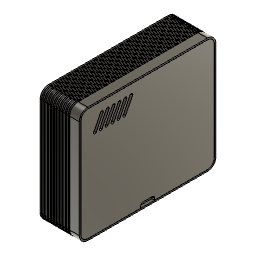
co2sensor_case (Autodesk Fusion 360 design; units mm, degrees)
Autodesk Fusion 360 part; units mm, degrees
note: some values were not read from the file. Set by a fixed rule: which sketch regions a step uses.
sketch "Front Layout" plane through (0, 0, 0) normal (1, 0, 0) x (0, 1, 0) in component "Front"
  line L0 (0, 0) -> (-45.7, 0)
  line L1 (-45.7, 0) -> (-45.7, 77.4)
  line L2 (-45.7, 77.4) -> (0, 77.4)
  line L3 (0, 77.4) -> (0, 0)
  line L4 (-48.7, 80.4) -> (0, 80.4)
  line L5 (0, 80.4) -> (0, -2)
  line L6 (0, -2) -> (-48.7, -2)
  line L7 (-48.7, -2) -> (-48.7, 80.4)
  line L8 (-42.2, 73.9) -> (0, 73.9)
  line L9 (0, 73.9) -> (0, 10.5)
  line L10 (0, 10.5) -> (-42.2, 10.5)
  line L11 (-42.2, 10.5) -> (-42.2, 73.9)
  dimension "d43" = 45.7
  dimension "d44" = 77.4
  dimension "d45" = 3
  dimension "d46" = 3
  dimension "d47" = 2
  dimension "d48" = 3.5
  dimension "d49" = 3.5
  dimension "d50" = 10.5
  constraint horizontal L0
  constraint vertical L1
  constraint horizontal L2
  constraint vertical L3
  constraint coincident L0.start L3.end
  constraint horizontal L4
  constraint vertical L5
  constraint horizontal L6
  constraint vertical L7
  constraint collinear L3 L5
  constraint horizontal L8
  constraint vertical L9
  constraint horizontal L10
  constraint vertical L11
  constraint collinear L3 L9
  measures "d43" distance of L0.start L0.end
  measures "d44" distance of L0.start L2.end
  measures "d45" distance of L2 L4
  measures "d46" distance of L1 L7
  measures "d47" distance of L0 L6
  measures "d48" distance of L2 L8
  measures "d49" distance of L1 L11
  measures "d50" distance of L0 L10
extrude "Extrude5" add sketch "Front Layout" along normal blind 28 makes body 1 in component "Front"
fillet "Fillet4" radius 6 2 edges at (14, -48.7, 80.4) (14, -48.7, -2) on bodies 1 in component "Front"
shell "Shell2" thickness 3 removed faces 2 at (18.6667, 0, 52.9333) at (28, -16.2333, 50.9333) on bodies 1 in component "Front"
extrude "Extrude6" cut sketch "Front Layout" along normal blind 3 contours L3 L5 L8 L9 L10 L11 bodies 1 in component "Front"
fillet "Fillet5" radius 3 2 edges at (1.5, -42.2, 73.9) (1.5, -42.2, 10.5) on bodies 1 in component "Front"
extrude "Extrude7" cut sketch "Front Layout" along normal blind 60 from surface at 3 contours L0 L1 L2 L3 L5 L8 L10 L11 bodies 1 in component "Front"
extrude "Extrude8" cut 1 faces at (3, -28.3, 3.5) along direction (-1, 0, 0) blind 1 on bodies 1 bodies 1 in component "Front"
sketch "Case Ribs" plane through (0, 0, 0) normal (-1, 0, 0) x (0, -1, 0) in component "Front"
  line L0 (39.2, 10.5) -> (0, 10.5)
  line L1 (0, 10.5) -> (0, -2)
  line L2 (0, -2) -> (42.7, -2)
  arc A0 (42.7, -2) -> (48.7, 4) centre (42.7, 4) ccw
  line L3 (48.7, 4) -> (48.7, 74.4)
  arc A1 (48.7, 74.4) -> (42.7, 80.4) centre (42.7, 74.4) ccw
  line L4 (42.7, 80.4) -> (0, 80.4)
  line L5 (0, 80.4) -> (0, 73.9)
  line L6 (0, 73.9) -> (39.2, 73.9)
  arc A2 (42.2, 70.9) -> (39.2, 73.9) centre (39.2, 70.9) ccw
  line L7 (42.2, 70.9) -> (42.2, 13.5)
  arc A3 (39.2, 10.5) -> (42.2, 13.5) centre (39.2, 13.5) ccw
  line L8 (0, -1.8) -> (42.7, -1.8)
  arc A4 (42.7, -1.8) -> (48.5, 4) centre (42.7, 4) ccw
  line L9 (48.5, 4) -> (48.5, 74.4)
  arc A5 (48.5, 74.4) -> (42.7, 80.2) centre (42.7, 74.4) ccw
  line L10 (42.7, 80.2) -> (0, 80.2)
  dimension "d67" = -0.2
extrude "Extrude9" cut sketch "Case Ribs" along normal blind 1 from surface at -2 contours L1 L2 A0 L3 A1 L4 L5 L8 A4 L9 A5 L10 bodies 1 in component "Front"
pattern_linear "R-Pattern1" count 10 spacing 2.1111 along (1, 0, 0) of "Extrude9" in component "Front"
sketch "Inlay Tabs" plane through (0, -45.7, 0) normal (0, 1, 0) x (-1, 0, 0) in component "Front"
  line L0 (-2, 77.4) -> (-28, 77.4)
  line L1 (-28, 77.4) -> (-28, 0)
  line L2 (-28, 0) -> (-2, 0)
  line L3 (-2, 0) -> (-2, 77.4)
  line L4 (-28, 71.4) -> (-2, 71.4)
  line L5 (-2, 71.4) -> (-2, 59.4)
  line L6 (-2, 59.4) -> (-28, 59.4)
  line L7 (-28, 59.4) -> (-28, 71.4)
  line L8 (-28, 18) -> (-2, 18)
  line L9 (-2, 18) -> (-2, 6)
  line L10 (-2, 6) -> (-28, 6)
  line L11 (-28, 6) -> (-28, 18)
  line L12 (-2, 70.9) -> (-2, 13.5)
  line L13 (-28, 77.4) -> (-2, 77.4)
  line L14 (-2, 0) -> (-28, 0)
  dimension "d81" = 12
  dimension "d82" = 12
  dimension "d83" = 6
  dimension "d84" = 6
  constraint horizontal L4
  constraint vertical L5
  constraint horizontal L6
  constraint vertical L7
  constraint horizontal L8
  constraint vertical L9
  constraint horizontal L10
  constraint vertical L11
  constraint collinear L5 L12
  constraint collinear L3 L9
  constraint collinear L1 L11
  constraint collinear L1 L7
  measures "d81" distance of L4.start L6.end
  measures "d82" distance of L8.start L10.end
  measures "d83" distance of L4 L13
  measures "d84" distance of L10 L14
extrude "Extrude11" cut sketch "Inlay Tabs" against normal blind 1 contours L1 L3 L4 L5 L6 L7 L12 | L1 L3 L8 L9 L10 L11 L12 bodies 1 in component "Front"
sketch "Backplate Groove" plane through (28, 0, 0) normal (1, 0, 0) x (0, 1, 0) in component "Front"
  line L0 (-45.7, 71.4) -> (-45.7, 77.4)
  line L1 (-45.7, 77.4) -> (0, 77.4)
  line L2 (0, 77.4) -> (0, 80.4)
  line L3 (0, 80.4) -> (-42.7, 80.4)
  arc A0 (-42.7, 80.4) -> (-48.7, 74.4) centre (-42.7, 74.4) ccw
  line L4 (-48.7, 74.4) -> (-48.7, 4)
  arc A1 (-48.7, 4) -> (-42.7, -2) centre (-42.7, 4) ccw
  line L5 (-42.7, -2) -> (0, -2)
  line L6 (0, -2) -> (0, 0)
  line L7 (0, 79.4) -> (-42.7, 79.4)
  arc A2 (-42.7, 79.4) -> (-47.7, 74.4) centre (-42.7, 74.4) ccw
  line L8 (-47.7, 74.4) -> (-47.7, 4)
  arc A3 (-47.7, 4) -> (-42.7, -1) centre (-42.7, 4) ccw
  line L9 (-42.7, -1) -> (0, -1)
  line L10 (0, 0) -> (-45.7, 0)
  line L11 (-45.7, 59.4) -> (-46.7, 59.4)
  line L12 (-46.7, 59.4) -> (-46.7, 71.4)
  line L13 (-46.7, 71.4) -> (-45.7, 71.4)
  line L14 (-45.7, 0) -> (-45.7, 6)
  line L15 (-45.7, 6) -> (-46.7, 6)
  line L16 (-46.7, 6) -> (-46.7, 18)
  line L17 (-46.7, 18) -> (-45.7, 18)
  line L18 (-45.7, 18) -> (-45.7, 59.4)
  dimension "d127" = -1
extrude "Extrude17" cut sketch "Backplate Groove" against normal blind 2.1 contours L0 L1 L2 L7 A2 L8 A3 L11 L12 L13 L14 L15 L16 L17 L18 | L6 A3 L9 L10 bodies 1 in component "Front"
ref_plane "WorkPlane1" through (0, 0, 41.1) normal (0, 0, 1) x (1, 0, 0) in component "Front"
sketch "Backplate Clip Indent" plane through (0, 0, 41.1) normal (0, 0, 1) x (1, 0, 0) in component "Front"
  line L0 (25.9, -45.7) -> (2, -45.7)
  line L1 (2, -45.7) -> (25.9, -45.7)
  line L2 (25.9, -45.7) -> (22.9, -45.7)
  line L3 (25.9, -45.7) -> (24.4, -47.2)
  line L4 (24.4, -47.2) -> (22.9, -45.7)
  dimension "d162" = 3
  constraint parallel L0 L2
  constraint perpendicular L3 L4
  constraint equal L3 L4
  constraint coincident L0.start L1.end
  measures "d162" distance of L0.start L2.end
extrude "Extrude19" cut sketch "Backplate Clip Indent" along normal blind 15 and the other way blind 15 bodies 1 in component "Front"
sketch "Inlay Layout" plane through (2, 0, 0) normal (1, 0, 0) x (0, 1, 0) in component "Inlay"
  arc A0 (-42.2, 13.5) -> (-39.2, 10.5) centre (-39.2, 13.5) ccw
  line L0 (-42.2, 13.5) -> (-42.2, 70.9)
  arc A1 (-39.2, 73.9) -> (-42.2, 70.9) centre (-39.2, 70.9) ccw
  line L1 (-39.2, 73.9) -> (0, 73.9)
  line L2 (0, 73.9) -> (0, 77.4)
  line L3 (0, 77.4) -> (-45.7, 77.4)
  line L4 (-45.7, 77.4) -> (-45.7, 71.4)
  line L5 (-45.7, 71.4) -> (-46.7, 71.4)
  line L6 (-46.7, 71.4) -> (-46.7, 59.4)
  line L7 (-46.7, 59.4) -> (-45.7, 59.4)
  line L8 (-45.7, 59.4) -> (-45.7, 18)
  line L9 (-45.7, 18) -> (-46.7, 18)
  line L10 (-46.7, 18) -> (-46.7, 6)
  line L11 (-46.7, 6) -> (-45.7, 6)
  line L12 (-45.7, 6) -> (-45.7, 0)
  line L13 (-45.7, 0) -> (0, 0)
  line L14 (0, 0) -> (0, 10.5)
  line L15 (0, 10.5) -> (-39.2, 10.5)
  line L16 (0, 77.2) -> (-45.5, 77.2)
  line L17 (-45.5, 77.2) -> (-45.5, 71.2)
  line L18 (-45.5, 71.2) -> (-46.5, 71.2)
  line L19 (-46.5, 71.2) -> (-46.5, 59.6)
  line L20 (-46.5, 59.6) -> (-45.5, 59.6)
  line L21 (-45.5, 59.6) -> (-45.5, 17.8)
  line L22 (-45.5, 17.8) -> (-46.5, 17.8)
  line L23 (-46.5, 17.8) -> (-46.5, 6.2)
  line L24 (-46.5, 6.2) -> (-45.5, 6.2)
  line L25 (-45.5, 6.2) -> (-45.5, 0.2)
  line L26 (-45.5, 0.2) -> (0, 0.2)
  line L27 (0, 77.2) -> (0, 0.2)
  line L28 (-45.5, 17.8) -> (-45.5, 6.2)
  line L29 (-45.5, 71.2) -> (-45.5, 59.6)
  circle A2 centre (-43.5, 75.2) radius 1
  circle A3 centre (-43.5, 75.2) radius 1.9
  circle A4 centre (-43.5, 2.2) radius 1
  circle A5 centre (-43.5, 2.2) radius 1.9
  dimension "d140" = -0.2
  dimension "d180" = 2
  dimension "d181" = 3.8
  dimension "d182" = 2
  dimension "d183" = 2
  dimension "d184" = 2
  dimension "d185" = 3.8
  dimension "d186" = 2
  dimension "d187" = 2
  constraint perpendicular L26 L27
  constraint concentric A2 A3
  constraint concentric A4 A5
  measures "d180" diameter of A2
  measures "d181" diameter of A3
  measures "d182" distance of L16 A2.centre
  measures "d183" distance of L17 A2.centre
  measures "d184" diameter of A4
  measures "d185" diameter of A5
  measures "d186" distance of L26 A4.centre
  measures "d187" distance of L25 A4.centre
extrude "Extrude3" add sketch "Inlay Layout" along normal blind 2 from surface at 1.5 separate body contours A0 L0 A1 L1 L15 L27 | A0 L0 A1 L1 L2 L14 L15 L16 L17 L21 L25 L26 L27 L28 L29 | A2 | A3 | A4 | A5 makes body 2 in component "Inlay"
extrude "Extrude4" add sketch "Inlay Layout" along normal blind 22.4 from surface at 1.5 contours L22 L23 L24 L28 | L18 L19 L20 L29 bodies 2 in component "Inlay"
sketch "Backplate Layout" plane through (28, 0, 0) normal (1, 0, 0) x (0, 1, 0) in component "Backplate"
  arc A0 (-47.7, 4) -> (-42.7, -1) centre (-42.7, 4) ccw
  line L0 (-47.7, 4) -> (-47.7, 74.4)
  arc A1 (-42.7, 79.4) -> (-47.7, 74.4) centre (-42.7, 74.4) ccw
  line L1 (-42.7, 79.4) -> (0, 79.4)
  line L2 (0, 79.4) -> (0, 80.4)
  line L3 (0, 80.4) -> (-42.7, 80.4)
  arc A2 (-42.7, 80.4) -> (-48.7, 74.4) centre (-42.7, 74.4) ccw
  line L4 (-48.7, 74.4) -> (-48.7, 4)
  arc A3 (-48.7, 4) -> (-42.7, -2) centre (-42.7, 4) ccw
  line L5 (-42.7, -2) -> (0, -2)
  line L6 (0, -2) -> (0, -1)
  line L7 (0, 79.3) -> (-42.7, 79.3)
  arc A4 (-42.7, 79.3) -> (-47.6, 74.4) centre (-42.7, 74.4) ccw
  line L8 (-47.6, 74.4) -> (-47.6, 4)
  arc A5 (-47.6, 4) -> (-42.7, -0.9) centre (-42.7, 4) ccw
  line L9 (-42.7, -0.9) -> (0, -0.9)
  line L10 (0, 79.3) -> (0, -0.9)
  line L11 (-47.6, 34) -> (-47.6, 45)
  line L12 (-35.032, -0.9) -> (-54, -0.9) construction
  line L13 (-30.185, 79.3) -> (-57.3808, 79.3) construction
  line L14 (-36.7056, 61.8528) -> (-31.7056, 71.8528)
  arc A6 (-31.7056, 71.8528) -> (-33.4944, 72.7472) centre (-32.6, 72.3) ccw
  line L15 (-33.4944, 72.7472) -> (-38.4944, 62.7472)
  arc A7 (-38.4944, 62.7472) -> (-36.7056, 61.8528) centre (-37.6, 62.3) ccw
  line L16 (-37.6, 62.3) -> (-32.6, 72.3) construction
  line L17 (-5, -0.9) -> (-5, 2.1)
  line L18 (-5, 2.1) -> (0, 2.1)
  line L19 (-29.2944, 72.7472) -> (-34.2944, 62.7472)
  line L20 (-32.5056, 61.8528) -> (-27.5056, 71.8528)
  arc A8 (-27.5056, 71.8528) -> (-29.2944, 72.7472) centre (-28.4, 72.3) ccw
  arc A9 (-34.2944, 62.7472) -> (-32.5056, 61.8528) centre (-33.4, 62.3) ccw
  line L21 (-25.0944, 72.7472) -> (-30.0944, 62.7472)
  line L22 (-28.3056, 61.8528) -> (-23.3056, 71.8528)
  arc A10 (-23.3056, 71.8528) -> (-25.0944, 72.7472) centre (-24.2, 72.3) ccw
  arc A11 (-30.0944, 62.7472) -> (-28.3056, 61.8528) centre (-29.2, 62.3) ccw
  line L23 (-20.8944, 72.7472) -> (-25.8944, 62.7472)
  line L24 (-24.1056, 61.8528) -> (-19.1056, 71.8528)
  arc A12 (-19.1056, 71.8528) -> (-20.8944, 72.7472) centre (-20, 72.3) ccw
  arc A13 (-25.8944, 62.7472) -> (-24.1056, 61.8528) centre (-25, 62.3) ccw
  line L25 (-16.6944, 72.7472) -> (-21.6944, 62.7472)
  line L26 (-19.9056, 61.8528) -> (-14.9056, 71.8528)
  arc A14 (-14.9056, 71.8528) -> (-16.6944, 72.7472) centre (-15.8, 72.3) ccw
  arc A15 (-21.6944, 62.7472) -> (-19.9056, 61.8528) centre (-20.8, 62.3) ccw
  line L27 (-12.4944, 72.7472) -> (-17.4944, 62.7472)
  line L28 (-15.7056, 61.8528) -> (-10.7056, 71.8528)
  arc A16 (-10.7056, 71.8528) -> (-12.4944, 72.7472) centre (-11.6, 72.3) ccw
  arc A17 (-17.4944, 62.7472) -> (-15.7056, 61.8528) centre (-16.6, 62.3) ccw
  line L29 (-2.6, 77.2) -> (-0.6, 77.2)
  line L30 (-0.6, 77.2) -> (-0.6, 57.2)
  line L31 (-0.6, 57.2) -> (-2.6, 57.2)
  line L32 (-2.6, 57.2) -> (-2.6, 77.2)
  line L33 (0, -1) -> (-42.7, -1)
  dimension "d147" = -1.1
  dimension "d194" = 2
  dimension "d195" = 10
  dimension "d196" = 7
  dimension "d197" = 15
  dimension "d198" = 17
  dimension "d211" = 5
  dimension "d212" = 3
  dimension "d219" = 21
  dimension "d220" = 0
  dimension "d221" = 2
  dimension "d222" = 20
  dimension "d223" = 45
  dimension "d224" = 2.1
  constraint perpendicular L9 L10
  constraint vertical L11
  constraint coincident L8 L11.end
  constraint coincident L9 L12.start
  constraint parallel L9 L12
  constraint coincident L7 L13.start
  constraint horizontal L13
  constraint tangent L14 A6
  constraint tangent A6 L15
  constraint parallel L14 L15
  constraint tangent L15 A7
  constraint tangent L14 A7
  constraint coincident L9 L17.start
  constraint perpendicular L9 L17
  constraint coincident L10 L18.end
  constraint perpendicular L10 L18
  constraint horizontal L29
  constraint vertical L30
  constraint horizontal L31
  constraint vertical L32
  measures "d194" diameter of A6
  measures "d195" distance of L8 A7.centre
  measures "d196" distance of L7 A6.centre
  measures "d197" distance of L8 A6.centre
  measures "d198" distance of L7 A7.centre
  measures "d211" distance of L17.end L18.end
  measures "d212" distance of L17.start L17.end
  measures "d221" distance of L29.start L29.end
  measures "d222" distance of L29.end L30.end
  measures "d223" distance of L8 L32
  measures "d224" distance of L7 L29
extrude "Extrude1" add sketch "Backplate Layout" against normal blind 2 separate body contours L7 A4 L8 A5 L9 L10 L11 L17 L18 | L9 L10 L17 L18 | L14 A6 L15 A7 | L19 L20 A8 A9 | L21 L22 A10 A11 | L23 L24 A12 A13 | L25 L26 A14 A15 | L27 L28 A16 A17 | L29 L30 L31 L32 makes body 3 in component "Backplate"
sketch "Backplate Clip" plane through (0, 0, 41.1) normal (0, 0, 1) x (1, 0, 0) in component "Backplate"
  line L0 (24.4, -47.2) -> (22.9, -45.7)
  line L1 (22.9, -45.7) -> (24.4, -47.2)
  line L2 (25.9, -45.7) -> (24.4, -47.2)
  line L3 (24.4, -47.2) -> (25.9, -45.7)
  line L4 (22.9, -45.5586) -> (24.4, -47.0586)
  line L5 (24.4, -47.0586) -> (25.803, -45.6556)
  line L6 (25.803, -45.6556) -> (26, -45.6556)
  line L7 (22.9, -45.5586) -> (25, -43.4586)
  line L8 (22.9, -45.5586) -> (25.8139, -45.5586) construction
  line L9 (25, -43.4586) -> (26, -43.4586)
  line L10 (26, -45.6556) -> (26, -43.4586)
  dimension "d167" = 0.1
  dimension "d168" = 0.1
  dimension "d226" = 45
  dimension "d227" = 1
  constraint perpendicular L4 L5
  constraint parallel L1 L4
  constraint equal L0 L4
  constraint horizontal L6
  constraint horizontal L8
  constraint horizontal L9
  constraint perpendicular L9 L10
  measures "d167" distance of L0 L4
  measures "d168" distance of L2 L5
  measures "d226" angle of L7 L8
  measures "d227" distance of L7.end L9.end
extrude "Extrude4'" add sketch "Backplate Clip" along normal blind 14 and the other way blind 14 bodies 3 in component "Backplate"
extrude "Extrude5'" add sketch "Inlay Layout" along normal blind 5 from surface at 1.5 contours A3 | A5 bodies 2 in component "Inlay"
mirror "Mirror2" about plane through (0, 0, 80.4) normal (0, 1, 0) of bodies 1 merged in component "Front"
mirror "Mirror1" about plane through (3.5, 0, 0.2) normal (0, 1, 0) of bodies 2 merged in component "Inlay"
extrude "Extrude7'" cut sketch "Backplate Layout" against normal blind 2 contours L9 L10 L17 L18 bodies 3 in component "Backplate"
fillet "Fillet1" radius 1.75 1 edges at (27, -5, 2.1) on bodies 3 in component "Backplate"
mirror "Mirror1'" about plane through (28, 0, 79.3) normal (0, 1, 0) of bodies 3 merged in component "Backplate"
extrude "Extrude5''" cut sketch "Backplate Layout" against normal blind 2 contours L14 A6 L15 A7 | L19 L20 A8 A9 | L21 L22 A10 A11 | L23 L24 A12 A13 | L25 L26 A14 A15 | L27 L28 A16 A17 bodies 3 in component "Backplate"
extrude "Extrude6'" add sketch "Backplate Layout" against normal blind 12 contours L29 L30 L31 L32 bodies 3 in component "Backplate"
component "Front" placed x (1, 0, 0) y (0, 1, 0) z (0, 0, 1) at (0, 0, 0)
component "Inlay" placed x (1, 0, 0) y (0, 1, 0) z (0, 0, 1) at (0, 0, 0)
component "Backplate" placed x (1, 0, 0) y (0, 1, 0) z (0, 0, 1) at (0, 0, 0)
